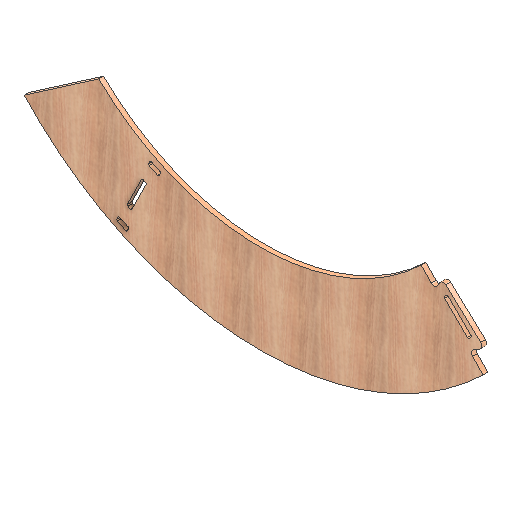
# Autodesk Inventor part: Platform E1
Saved by Autodesk Inventor 2021 (Build 250183000, 183)
## iProperties
Created: 2020-05-09
Part Number: Platform E1
Material: Wood (Birch)
Document SubType Name: Modeling
Designer: Dan Wikman
Density: 0.55 g/cm^3
Appearance: Birch - Natural Polished
Mass: 5553.92 g
Surface Area: 12101.6 cm^2
Volume: 10098 cm^3
Autodesk Inventor part; units mm, degrees
ref_plane "YZ Plane" through (0, 0, 0) normal (1, 0, 0) x (0, 1, 0)
ref_plane "XZ Plane" through (0, 0, 0) normal (0, 1, 0) x (-1, 0, 0)
ref_plane "XY Plane" through (0, 0, 0) normal (0, 0, 1) x (1, 0, 0)
sketch "CONTOURS" plane through (0, 0, 0) normal (0, 0, 1) x (1, 0, 0)
  arc A0 (1567.8979, 1059.3694) -> (1592.5572, 1062.5103) centre (1579.0574, 1070.1265) ccw
  line L0 (1592.5572, 1062.5103) -> (1600.8567, 1077.2212)
  arc A1 (1623.3344, 1080.7382) -> (1600.8567, 1077.2212) centre (1613.4855, 1070.0964) ccw
  line L1 (1623.3344, 1080.7382) -> (1755.4047, 958.5078)
  arc A2 (1752.9302, 935.3813) -> (1755.4047, 958.5078) centre (1745.5558, 947.866) ccw
  line L2 (1752.9302, 935.3813) -> (1728.0763, 920.7006)
  arc A3 (1728.0763, 920.7006) -> (1724.7998, 896.5978) centre (1735.9593, 907.3549) ccw
  line L3 (1724.7998, 896.5978) -> (1764.2337, 855.6886)
  arc A4 (25.6661, 904.4304) -> (1764.2337, 855.6886) centre (918.8737, 1733.3946) ccw
  line L4 (25.6661, 904.4304) -> (308.0876, 1099.0382)
  arc A5 (308.0876, 1099.0382) -> (1529.6596, 1099.0382) centre (918.8736, 1733.3944) ccw
  line L5 (1529.6596, 1099.0382) -> (1567.8979, 1059.3694)
  dimension "d1" = 1218.6064
  dimension "d3" = 880.6062
  constraints: 12 end point, 12 point on circle, 6 centre point
  measures "d1" radius of A4
  measures "d3" radius of A5
sketch "HOLES" plane through (0, 0, 0) normal (0, 0, 1) x (1, 0, 0)
  line L0 (376.9652, 673.5139) -> (381.8614, 683.3642)
  arc A0 (387.2238, 685.1656) -> (381.8614, 683.3642) centre (385.4433, 681.5837) ccw
  line L1 (387.2238, 685.1656) -> (419.4609, 669.1416)
  arc A1 (421.2623, 663.7792) -> (419.4609, 669.1416) centre (417.6804, 665.5597) ccw
  arc A2 (1631.4879, 1048.1109) -> (1625.8313, 1048.0547) centre (1628.6877, 1045.2545) ccw
  line L2 (1718.6644, 957.049) -> (1710.9639, 949.1939)
  arc A3 (1705.3073, 949.1377) -> (1710.9639, 949.1939) centre (1708.1075, 951.9941) ccw
  line L3 (1705.3073, 949.1377) -> (1618.1871, 1034.543)
  arc A4 (1618.1309, 1040.1996) -> (1618.1871, 1034.543) centre (1620.9873, 1037.3994) ccw
  line L4 (1618.1309, 1040.1996) -> (1625.8313, 1048.0547)
  line L5 (1631.4879, 1048.1109) -> (1718.6081, 962.7056)
  arc A5 (1718.6644, 957.049) -> (1718.6081, 962.7056) centre (1715.808, 959.8492) ccw
  line L6 (497.3235, 915.6504) -> (502.2197, 925.5006)
  arc A6 (507.5821, 927.3021) -> (502.2197, 925.5006) centre (505.8016, 923.7202) ccw
  line L7 (507.5821, 927.3021) -> (539.8192, 911.2781)
  arc A7 (541.6206, 905.9157) -> (539.8192, 911.2781) centre (538.0387, 907.6962) ccw
  line L8 (416.4201, 741.8384) -> (470.5996, 851.148)
  arc A8 (531.362, 894.264) -> (536.7244, 896.0655) centre (533.1425, 897.8459) ccw
  line L9 (531.362, 894.264) -> (499.1249, 910.2881)
  arc A9 (497.3235, 915.6504) -> (499.1249, 910.2881) centre (500.9054, 913.87) ccw
  line L10 (479.5438, 851.1791) -> (485.8157, 848.0705)
  arc A10 (487.6232, 842.7102) -> (485.8157, 848.0705) centre (484.0393, 844.4865) ccw
  line L11 (487.6232, 842.7102) -> (433.4437, 733.4006)
  arc A11 (428.0834, 731.5931) -> (433.4437, 733.4006) centre (429.8598, 735.177) ccw
  line L12 (428.0834, 731.5931) -> (418.2276, 736.4781)
  arc A12 (416.4201, 741.8384) -> (418.2276, 736.4781) centre (420.004, 740.062) ccw
  line L13 (541.6206, 905.9157) -> (536.7244, 896.0655)
  arc A13 (475.9599, 852.9555) -> (470.5996, 851.148) centre (474.1835, 849.3716) ccw
  line L14 (475.9599, 852.9555) -> (479.5438, 851.1791)
  line L15 (421.2623, 663.7792) -> (416.3661, 653.929)
  arc A14 (411.0038, 652.1276) -> (416.3661, 653.929) centre (412.7842, 655.7095) ccw
  line L16 (411.0038, 652.1276) -> (378.7667, 668.1516)
  arc A15 (376.9652, 673.5139) -> (378.7667, 668.1516) centre (380.5471, 671.7335) ccw
  dimension "d5" = 0.065
  dimension "d7" = 0.065
  constraints: 34 end point, 32 point on circle, 16 centre point
  measures "d5" angle of L15 L11
  measures "d7" angle of L8 L0
sketch "LETTERS" plane through (0, 0, 0) normal (0, 0, 1) x (1, 0, 0)
  line L0 (544.6299, 751.705) -> (554.564, 747.8187)
  line L1 (561.8694, 755.3769) -> (548.1913, 760.7277)
  line L2 (548.1913, 760.7277) -> (540.975, 742.2812)
  line L3 (540.975, 742.2812) -> (554.6531, 736.9303)
  constraints: 8 end point, 2 parallel, 1 perpendicular
extrude "Extrusion3" add sketch "CONTOURS" along normal blind 18
extrude "Extrusion4" cut sketch "HOLES" along normal blind 18
body "Solid2"
